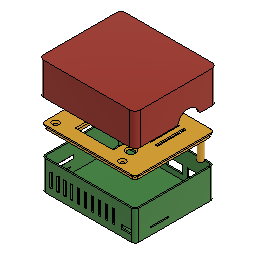
Raspi Zero 2W Case Battery V1 (Autodesk Fusion 360 design; units mm, degrees)
Autodesk Fusion 360 part; units mm, degrees
sketch "Skizze1" plane through (0, 0, 0) normal (0, 0, 1) x (1, 0, 0)
  line L0 (0, 0) -> (78.8, 0) construction
  line L1 (78.8, 0) -> (78.8, 62.5) construction
  line L2 (78.8, 62.5) -> (0, 62.5) construction
  line L3 (0, 62.5) -> (0, 0) construction
  line L4 (2, 65) -> (76.8, 65)
  line L5 (78.8, 63) -> (78.8, 0.5)
  line L6 (76.8, -1.5) -> (2, -1.5)
  line L7 (0, 0.5) -> (0, 63)
  circle A0 centre (75.3, 59) radius 1.5
  circle A1 centre (4.8, 59) radius 1.5
  circle A2 centre (4.8, 3.5) radius 1.5
  circle A3 centre (62.8, 3.5) radius 1.5
  circle A4 centre (4.8, 26.5) radius 1.5
  circle A5 centre (62.8, 26.5) radius 1.5
  circle A6 centre (4.8, 59) radius 2.5
  circle A7 centre (75.3, 59) radius 2.5
  circle A8 centre (4.8, 3.5) radius 2.5
  circle A9 centre (62.8, 3.5) radius 2.5
  arc A10 (78.8, 63) -> (76.8, 65) centre (76.8, 63) ccw
  arc A11 (2, 65) -> (0, 63) centre (2, 63) ccw
  arc A12 (0, 0.5) -> (2, -1.5) centre (2, 0.5) ccw
  arc A13 (76.8, -1.5) -> (78.8, 0.5) centre (76.8, 0.5) ccw
  line L8 (76.8, -2.7) -> (2, -2.7)
  arc A14 (-1.2, 0.5) -> (2, -2.7) centre (2, 0.5) ccw
  line L9 (-1.2, 0.5) -> (-1.2, 63)
  arc A15 (2, 66.2) -> (-1.2, 63) centre (2, 63) ccw
  line L10 (2, 66.2) -> (76.8, 66.2)
  arc A16 (80, 63) -> (76.8, 66.2) centre (76.8, 63) ccw
  line L11 (80, 63) -> (80, 0.5)
  arc A17 (76.8, -2.7) -> (80, 0.5) centre (76.8, 0.5) ccw
  dimension "d1" = 78.8
  dimension "d2" = 62.5
  dimension "d7" = 66.5
  dimension "d8" = 78.8
  dimension "d9" = 78.8
  dimension "d10" = 2.5
  dimension "d11" = 3
  dimension "d13" = 3.5
  dimension "d15" = 3
  dimension "d16" = 4.8
  dimension "d18" = 3.5
  dimension "d19" = 3.5
  dimension "d21" = 3
  dimension "d22" = 3.5
  dimension "d23" = 4.8
  dimension "d24" = 3
  dimension "d25" = 3.5
  dimension "d26" = 58
  dimension "d29" = 3
  dimension "d30" = 23
  dimension "d31" = 4.8
  dimension "d32" = 3
  dimension "d33" = 58
  dimension "d34" = 23
  dimension "d44" = 5
  dimension "d45" = 5
  dimension "d46" = 5
  dimension "d47" = 5
  dimension "d50" = 2
  dimension "d112" = 70.5
  constraint horizontal L0
  constraint vertical L1
  constraint horizontal L2
  constraint vertical L3
  constraint coincident L0.start L3.end
  constraint horizontal L4
  constraint vertical L5
  constraint horizontal L6
  constraint vertical L7
  constraint concentric A1 A6
  constraint concentric A0 A7
  constraint concentric A2 A8
  constraint concentric A3 A9
  constraint tangent L4 A10
  constraint tangent L5 A10
  constraint tangent L4 A11
  constraint tangent L7 A11
  constraint equal A10 A11
  constraint tangent L6 A12
  constraint tangent L7 A12
  constraint equal A10 A12
  constraint tangent L5 A13
  constraint tangent L6 A13
  constraint equal A10 A13
  measures "d1" distance of L0.start L0.end
  measures "d2" distance of L0.start L2.end
  measures "d7" distance of L4 L6
  measures "d8" distance of L5 L7
  measures "d9" distance of L3 L5
  measures "d10" distance of L2 L4
  measures "d11" diameter of A0
  measures "d13" distance of L5 A0.centre
  measures "d15" diameter of A1
  measures "d16" distance of L7 A1.centre
  measures "d18" distance of L2 A1.centre
  measures "d19" distance of L2 A0.centre
  measures "d21" diameter of A2
  measures "d22" distance of L0 A2.centre
  measures "d23" distance of L7 A2.centre
  measures "d24" diameter of A3
  measures "d25" distance of L0 A3.centre
  measures "d26" distance of A2.centre A3.centre
  measures "d29" diameter of A4
  measures "d30" vertical distance of A2.centre A4.centre
  measures "d31" distance of L7 A4.centre
  measures "d32" diameter of A5
  measures "d33" horizontal distance of A4.centre A5.centre
  measures "d34" distance of A3.centre A5.centre
  measures "d44" diameter of A6
  measures "d45" diameter of A7
  measures "d46" diameter of A8
  measures "d47" diameter of A9
  measures "d50" radius of A10
  measures "d112" distance of A1.centre A0.centre
extrude "Extrusion1" add sketch "Skizze1" against normal blind 1.2 contours L4 L5 L6 L7 A10 A11 A12 A13 | A0 | A1 | A2 | A3 | A4 | A5 | A6 | A7 | A8 | A9 | L8 A14 L9 A15 L10 A16 L11 A17 makes body 1
extrude "Extrusion2" add sketch "Skizze1" along normal blind 24.5 contours L8 A14 L9 A15 L10 A16 L11 A17 bodies 1
extrude "Extrusion3" add sketch "Skizze1" along normal blind 3 contours A6 | A7 | A8 | A9 bodies 1
extrude "Extrusion4" cut sketch "Skizze1" against normal blind 1.2 contours A0 | A1 | A2 | A3 bodies 1
chamfer "Fase1" distance 1.4 angle 45 4 edges at (61.4015, 2.9576, -1.2) (3.4015, 2.9576, -1.2) (3.4015, 58.4576, -1.2) (73.9015, 58.4576, -1.2) on bodies 1
ref_plane "Arbeitsebene1" through (82, 31.75, 11.65) normal (1, 0, 0) x (0, -1, 0)
sketch "Skizze2" plane through (82, 0, 0) normal (1, 0, 0) x (0, 1, 0)
  line L0 (11, 5.5) -> (26, 5.5)
  line L1 (26, 5.5) -> (26, 4.5)
  line L2 (26, 4.5) -> (11, 4.5)
  line L3 (11, 4.5) -> (11, 5.5)
  line L4 (7, 19.5) -> (8.5, 19.5)
  line L5 (8.5, 19.5) -> (8.5, 14.5)
  line L6 (8.5, 14.5) -> (7, 14.5)
  line L7 (7, 14.5) -> (7, 19.5)
  dimension "d65" = 15
  dimension "d66" = 1
  dimension "d68" = 11
  dimension "d69" = 4.5
  dimension "d109" = 1.5
  dimension "d110" = 5
  dimension "d111" = 14.5
  dimension "d119" = 7
  constraint horizontal L0
  constraint vertical L1
  constraint horizontal L2
  constraint vertical L3
  constraint horizontal L4
  constraint vertical L5
  constraint horizontal L6
  constraint vertical L7
  measures "d65" distance of L1 L3
  measures "d66" distance of L0 L2
  measures "d68" distance of origin L3
  measures "d69" distance of origin L2
  measures "d109" distance of L4.start L4.end
  measures "d110" distance of L4.start L6.end
  measures "d111" distance of origin L6
  measures "d119" distance of origin L7
extrude "Extrusion5" cut sketch "Skizze2" against normal blind 3.2 contours L0 L1 L2 L3 bodies 1
ref_plane "Arbeitsebene2" through (-3.2, 31.75, 11.65) normal (-1, 0, 0) x (0, 1, 0)
sketch "Skizze3" plane through (-3.2, 0, 0) normal (-1, 0, 0) x (0, -1, 0)
  line L0 (-21, 5.5) -> (-8, 5.5)
  line L1 (-8, 5.5) -> (-8, 4.5)
  line L2 (-8, 4.5) -> (-21, 4.5)
  line L3 (-21, 4.5) -> (-21, 5.5)
  line L4 (-63, 0) -> (-0.5, 0)
  line L5 (-24, 13) -> (-11, 13)
  line L6 (-11, 13) -> (-11, 10)
  line L7 (-11, 10) -> (-24, 10)
  line L8 (-24, 10) -> (-24, 13)
  dimension "d73" = 13
  dimension "d74" = 1
  dimension "d75" = 8
  dimension "d76" = 4.5
  dimension "d77" = 13
  dimension "d78" = 3
  dimension "d79" = 11
  dimension "d80" = 10
  constraint horizontal L0
  constraint vertical L1
  constraint horizontal L2
  constraint vertical L3
  constraint horizontal L5
  constraint vertical L6
  constraint horizontal L7
  constraint vertical L8
  measures "d73" distance of L0.start L0.end
  measures "d74" distance of L0 L2
  measures "d75" distance of origin L1
  measures "d76" distance of L2 L4
  measures "d77" distance of L6 L8
  measures "d78" distance of L5 L7
  measures "d79" distance of origin L6
  measures "d80" distance of L4 L7
extrude "Extrusion6" cut sketch "Skizze3" against normal blind 3.2 bodies 1
chamfer "Fase4" distance 1 angle 45 4 edges at (-1.2, 17.5, 13) (-1.2, 11, 11.5) (-1.2, 17.5, 10) (-1.2, 24, 11.5) on bodies 1
ref_plane "Arbeitsebene3" through (39.4, -4.7, 11.65) normal (0, -1, 0) x (-1, 0, 0)
sketch "Skizze4" plane through (0, -4.7, 0) normal (0, -1, 0) x (-1, 0, 0)
  line L0 (-76.8, -8) -> (-67.8, -8)
  line L1 (-67.8, -8) -> (-67.8, -4.5)
  line L2 (-67.8, -4.5) -> (-76.8, -4.5)
  line L3 (-76.8, -4.5) -> (-76.8, -8)
  line L4 (-6, -16.5) -> (-8, -16.5)
  line L5 (-8, -16.5) -> (-8, -4.5)
  line L6 (-8, -4.5) -> (-6, -4.5)
  line L7 (-6, -4.5) -> (-6, -16.5)
  line L8 (-12, -4.5) -> (-12, -16.5)
  line L9 (-14, -4.5) -> (-12, -4.5)
  line L10 (-14, -16.5) -> (-14, -4.5)
  line L11 (-12, -16.5) -> (-14, -16.5)
  line L12 (-18, -4.5) -> (-18, -16.5)
  line L13 (-20, -4.5) -> (-18, -4.5)
  line L14 (-20, -16.5) -> (-20, -4.5)
  line L15 (-18, -16.5) -> (-20, -16.5)
  line L16 (-24, -4.5) -> (-24, -16.5)
  line L17 (-26, -4.5) -> (-24, -4.5)
  line L18 (-26, -16.5) -> (-26, -4.5)
  line L19 (-24, -16.5) -> (-26, -16.5)
  line L20 (-30, -4.5) -> (-30, -16.5)
  line L21 (-32, -4.5) -> (-30, -4.5)
  line L22 (-32, -16.5) -> (-32, -4.5)
  line L23 (-30, -16.5) -> (-32, -16.5)
  line L24 (-36, -4.5) -> (-36, -16.5)
  line L25 (-38, -4.5) -> (-36, -4.5)
  line L26 (-38, -16.5) -> (-38, -4.5)
  line L27 (-36, -16.5) -> (-38, -16.5)
  line L28 (-42, -4.5) -> (-42, -16.5)
  line L29 (-44, -4.5) -> (-42, -4.5)
  line L30 (-44, -16.5) -> (-44, -4.5)
  line L31 (-42, -16.5) -> (-44, -16.5)
  line L32 (-48, -4.5) -> (-48, -16.5)
  line L33 (-50, -4.5) -> (-48, -4.5)
  line L34 (-50, -16.5) -> (-50, -4.5)
  line L35 (-48, -16.5) -> (-50, -16.5)
  line L36 (-54, -4.5) -> (-54, -16.5)
  line L37 (-56, -4.5) -> (-54, -4.5)
  line L38 (-56, -16.5) -> (-56, -4.5)
  line L39 (-54, -16.5) -> (-56, -16.5)
  line L40 (-60, -4.5) -> (-60, -16.5)
  line L41 (-62, -4.5) -> (-60, -4.5)
  line L42 (-62, -16.5) -> (-62, -4.5)
  line L43 (-60, -16.5) -> (-62, -16.5)
  dimension "d84" = 9
  dimension "d85" = 3.5
  dimension "d86" = 76.8
  dimension "d87" = 4.5
  dimension "d171" = 2
  dimension "d172" = 12
  dimension "d173" = 4.5
  dimension "d176" = -6
  dimension "d177" = 0
  dimension "d178" = 6
  constraint horizontal L0
  constraint vertical L1
  constraint horizontal L2
  constraint vertical L3
  constraint horizontal L4
  constraint vertical L5
  constraint horizontal L6
  constraint vertical L7
  measures "d84" distance of L0.start L0.end
  measures "d85" distance of L0 L2
  measures "d86" distance of origin L3
  measures "d87" distance of origin L2
  measures "d171" distance of L5 L7
  measures "d172" distance of L4 L6
  measures "d173" distance of origin L6
  measures "d178" distance of origin L7
extrude "Extrusion7" cut sketch "Skizze4" against normal blind 3.2 bodies 1
ref_plane "Arbeitsebene4" through (39.4, 68.2, 11.65) normal (0, 1, 0) x (1, 0, 0)
sketch "Skizze5" plane through (0, 68.2, 0) normal (0, 1, 0) x (1, 0, 0)
  line L0 (76.8, 0) -> (2, 0)
  line L1 (35.8, -11.5) -> (21.8, -11.5)
  line L2 (21.8, -11.5) -> (21.8, -4.5)
  line L3 (21.8, -4.5) -> (35.8, -4.5)
  line L4 (35.8, -4.5) -> (35.8, -11.5)
  line L5 (53.8, -11.5) -> (39.8, -11.5)
  line L6 (39.8, -11.5) -> (39.8, -4.5)
  line L7 (39.8, -4.5) -> (53.8, -4.5)
  line L8 (53.8, -4.5) -> (53.8, -11.5)
  line L9 (71.8, -11.5) -> (57.8, -11.5)
  line L10 (57.8, -11.5) -> (57.8, -4.5)
  line L11 (57.8, -4.5) -> (71.8, -4.5)
  line L12 (71.8, -4.5) -> (71.8, -11.5)
  line L13 (13.4, -13.3) -> (10.4, -13.3)
  line L14 (10.4, -13.3) -> (10.4, -3.3)
  line L15 (10.4, -3.3) -> (13.4, -3.3)
  line L16 (13.4, -3.3) -> (13.4, -13.3)
  line L17 (11.9, -49) -> (11.9, 25) construction
  line L18 (91, -8.3) -> (-18, -8.3) construction
  line L19 (-1.2, 1.2) -> (-1.2, -24.5)
  line L20 (2, 1.2) -> (76.8, 1.2)
  circle A0 centre (11.9, -8.3) radius 2.25
  dimension "d94" = 14
  dimension "d95" = 7
  dimension "d96" = 11.5
  dimension "d97" = 21.8
  dimension "d98" = 7
  dimension "d99" = 11.5
  dimension "d100" = 14
  dimension "d101" = 18
  dimension "d102" = 7
  dimension "d103" = 14
  dimension "d104" = 11.5
  dimension "d105" = 18
  dimension "d114" = 10
  dimension "d115" = 3
  dimension "d124" = 4.5
  dimension "d125" = 11.9
  dimension "d126" = 8.3
  constraint horizontal L1
  constraint vertical L2
  constraint horizontal L3
  constraint vertical L4
  constraint horizontal L5
  constraint vertical L6
  constraint horizontal L7
  constraint vertical L8
  constraint horizontal L9
  constraint vertical L10
  constraint horizontal L11
  constraint vertical L12
  constraint horizontal L13
  constraint vertical L14
  constraint horizontal L15
  constraint vertical L16
  constraint perpendicular L0 L17
  constraint perpendicular L6 L18
  constraint coincident L18 A0.centre
  constraint coincident L17 A0.centre
  constraint symmetric L13 L15 L18
  constraint symmetric L14 L16 L17
  measures "d94" distance of L1.start L1.end
  measures "d95" distance of L1.start L3.end
  measures "d96" distance of L0 L1
  measures "d97" distance of origin L2
  measures "d98" distance of L5 L7
  measures "d99" distance of L0 L5
  measures "d100" distance of L6 L8
  measures "d101" distance of L2 L6
  measures "d102" distance of L9 L11
  measures "d103" distance of L10 L12
  measures "d104" distance of L0 L9
  measures "d105" distance of L6 L10
  measures "d114" distance of L13 L15
  measures "d115" distance of L14 L16
  measures "d124" diameter of A0
  measures "d125" distance of origin L17
  measures "d126" distance of origin L18
extrude "Extrusion8" cut sketch "Skizze5" against normal blind 3.2 bodies 1
chamfer "Fase6" distance 1 angle 45 8 edges at (11.9, 66.2, 13.3) (10.4, 66.2, 11.6385) (9.65, 66.2, 8.3) (10.4, 66.2, 4.9615) (11.9, 66.2, 3.3) (13.4, 66.2, 4.9615) (14.15, 66.2, 8.3) (13.4, 66.2, 11.6385) on bodies 1
ref_plane "Arbeitsebene5" through (39.4, 31.75, 28.5) normal (0, 0, 1) x (1, 0, 0)
sketch "Skizze6" plane through (0, 0, 28.5) normal (0, 0, 1) x (1, 0, 0)
  arc A0 (0, 0.5) -> (2, -1.5) centre (2, 0.5) ccw construction
  line L0 (0, 0.5) -> (0, 63) construction
  arc A1 (2, 65) -> (0, 63) centre (2, 63) ccw construction
  line L1 (2, 65) -> (76.8, 65) construction
  arc A2 (78.8, 63) -> (76.8, 65) centre (76.8, 63) ccw construction
  line L2 (78.8, 63) -> (78.8, 0.5) construction
  arc A3 (76.8, -1.5) -> (78.8, 0.5) centre (76.8, 0.5) ccw construction
  line L3 (76.8, -1.5) -> (2, -1.5) construction
  arc A4 (-1.2, 0.5) -> (2, -2.7) centre (2, 0.5) ccw construction
  line L4 (2, -2.7) -> (76.8, -2.7) construction
  arc A5 (76.8, -2.7) -> (80, 0.5) centre (76.8, 0.5) ccw construction
  line L5 (80, 0.5) -> (80, 63) construction
  arc A6 (80, 63) -> (76.8, 66.2) centre (76.8, 63) ccw construction
  line L6 (76.8, 66.2) -> (2, 66.2) construction
  arc A7 (2, 66.2) -> (-1.2, 63) centre (2, 63) ccw construction
  line L7 (-1.2, 63) -> (-1.2, 0.5) construction
  circle A8 centre (4.8, 3.5) radius 1.5
  circle A9 centre (62.8, 3.5) radius 1.5
  circle A10 centre (75.3, 59) radius 1.5
  circle A11 centre (4.8, 59) radius 1.5
  arc A12 (2, 64.95) -> (0.05, 63) centre (2, 63) ccw
  line L8 (0.05, 0.5) -> (0.05, 63)
  arc A13 (0.05, 0.5) -> (2, -1.45) centre (2, 0.5) ccw
  line L9 (76.8, -1.45) -> (2, -1.45)
  arc A14 (76.8, -1.45) -> (78.75, 0.5) centre (76.8, 0.5) ccw
  line L10 (78.75, 63) -> (78.75, 0.5)
  arc A15 (78.75, 63) -> (76.8, 64.95) centre (76.8, 63) ccw
  line L11 (2, 64.95) -> (76.8, 64.95)
  arc A16 (2, 63.75) -> (1.25, 63) centre (2, 63) ccw
  line L12 (1.25, 0.5) -> (1.25, 63)
  arc A17 (1.25, 0.5) -> (2, -0.25) centre (2, 0.5) ccw
  line L13 (76.8, -0.25) -> (2, -0.25)
  arc A18 (76.8, -0.25) -> (77.55, 0.5) centre (76.8, 0.5) ccw
  line L14 (77.55, 63) -> (77.55, 0.5)
  arc A19 (77.55, 63) -> (76.8, 63.75) centre (76.8, 63) ccw
  line L15 (2, 63.75) -> (76.8, 63.75)
  arc A20 (2, 66.2) -> (-1.2, 63) centre (2, 63) ccw
  line L16 (-1.2, 0.5) -> (-1.2, 63)
  arc A21 (-1.2, 0.5) -> (2, -2.7) centre (2, 0.5) ccw
  line L17 (76.8, -2.7) -> (2, -2.7)
  arc A22 (76.8, -2.7) -> (80, 0.5) centre (76.8, 0.5) ccw
  line L18 (80, 63) -> (80, 0.5)
  arc A23 (80, 63) -> (76.8, 66.2) centre (76.8, 63) ccw
  line L19 (2, 66.2) -> (76.8, 66.2)
  circle A24 centre (4.8, 3.5) radius 2.5
  circle A25 centre (4.8, 59) radius 2.5
  circle A26 centre (75.3, 59) radius 2.5
  circle A27 centre (62.8, 3.5) radius 2.5
  circle A28 centre (58.55, 15.25) radius 3
  line L20 (18.3, 25) -> (49.3, 25)
  line L21 (49.3, 25) -> (49.3, 9)
  line L22 (49.3, 9) -> (18.3, 9)
  line L23 (18.3, 9) -> (18.3, 25)
  line L24 (50.5, 26.2) -> (50.5, 7.8)
  line L25 (50.5, 7.8) -> (17.1, 7.8)
  line L26 (17.1, 7.8) -> (17.1, 26.2)
  line L27 (17.1, 26.2) -> (50.5, 26.2)
  line L28 (10.8, 54.95) -> (12.8, 54.95)
  line L29 (12.8, 54.95) -> (12.8, 29.95)
  line L30 (12.8, 29.95) -> (10.8, 29.95)
  line L31 (10.8, 29.95) -> (10.8, 54.95)
  line L32 (16.8, 54.95) -> (18.8, 54.95)
  line L33 (16.8, 29.95) -> (16.8, 54.95)
  line L34 (18.8, 54.95) -> (18.8, 29.95)
  line L35 (18.8, 29.95) -> (16.8, 29.95)
  line L36 (22.8, 54.95) -> (24.8, 54.95)
  line L37 (22.8, 29.95) -> (22.8, 54.95)
  line L38 (24.8, 54.95) -> (24.8, 29.95)
  line L39 (24.8, 29.95) -> (22.8, 29.95)
  line L40 (28.8, 54.95) -> (30.8, 54.95)
  line L41 (28.8, 29.95) -> (28.8, 54.95)
  line L42 (30.8, 54.95) -> (30.8, 29.95)
  line L43 (30.8, 29.95) -> (28.8, 29.95)
  line L44 (34.8, 54.95) -> (36.8, 54.95)
  line L45 (34.8, 29.95) -> (34.8, 54.95)
  line L46 (36.8, 54.95) -> (36.8, 29.95)
  line L47 (36.8, 29.95) -> (34.8, 29.95)
  line L48 (40.8, 54.95) -> (42.8, 54.95)
  line L49 (40.8, 29.95) -> (40.8, 54.95)
  line L50 (42.8, 54.95) -> (42.8, 29.95)
  line L51 (42.8, 29.95) -> (40.8, 29.95)
  line L52 (46.8, 54.95) -> (48.8, 54.95)
  line L53 (46.8, 29.95) -> (46.8, 54.95)
  line L54 (48.8, 54.95) -> (48.8, 29.95)
  line L55 (48.8, 29.95) -> (46.8, 29.95)
  line L56 (52.8, 54.95) -> (54.8, 54.95)
  line L57 (52.8, 29.95) -> (52.8, 54.95)
  line L58 (54.8, 54.95) -> (54.8, 29.95)
  line L59 (54.8, 29.95) -> (52.8, 29.95)
  line L60 (58.8, 54.95) -> (60.8, 54.95)
  line L61 (58.8, 29.95) -> (58.8, 54.95)
  line L62 (60.8, 54.95) -> (60.8, 29.95)
  line L63 (60.8, 29.95) -> (58.8, 29.95)
  line L64 (64.8, 54.95) -> (66.8, 54.95)
  line L65 (64.8, 29.95) -> (64.8, 54.95)
  line L66 (66.8, 54.95) -> (66.8, 29.95)
  line L67 (66.8, 29.95) -> (64.8, 29.95)
  circle A29 centre (75.3, 59) radius 1.2
  circle A30 centre (4.8, 59) radius 1.2
  dimension "d130" = 0.05
  dimension "d131" = 1.25
  dimension "d143" = 6
  dimension "d144" = 11.75
  dimension "d145" = 4.25
  dimension "d149" = 31
  dimension "d150" = 16
  dimension "d151" = 5.5
  dimension "d152" = 13.5
  dimension "d159" = 10
  dimension "d160" = 10.75
  dimension "d163" = 6
  dimension "d164" = 0
  dimension "d165" = 56
  dimension "d179" = 2.4
  dimension "d180" = 2.4
  constraint horizontal L20
  constraint vertical L21
  constraint horizontal L22
  constraint vertical L23
  constraint horizontal L28
  constraint vertical L29
  constraint horizontal L30
  constraint vertical L31
  constraint concentric A10 A29
  constraint concentric A11 A30
  measures "d143" diameter of A28
  measures "d144" vertical distance of A9.centre A28.centre
  measures "d145" horizontal distance of A9.centre A28.centre
  measures "d149" distance of L20.start L20.end
  measures "d150" distance of L20.start L22.end
  measures "d151" distance of A9.centre L22
  measures "d152" distance of A9.centre L21
  measures "d159" distance of L11 L28
  measures "d160" distance of L8 L31
  measures "d165" distance of L31 L66
  measures "d179" diameter of A29
  measures "d180" diameter of A30
extrude "Extrusion9" add sketch "Skizze6" along normal blind 1.2 separate body contours A8 | A9 | A10 | A11 | A12 L8 A13 L9 A14 L10 A15 L11 | A16 L12 A17 L13 A18 L14 A19 L15 A26 | L14 A26 | L14 A26 | A20 L16 A21 L17 A22 L18 A23 L19 | A24 | A25 | A27 | A28 | L20 L21 L22 L23 | L24 L25 L26 L27 | L28 L29 L30 L31 | L32 L33 L34 L35 | L36 L37 L38 L39 | L40 L41 L42 L43 | L44 L45 L46 L47 | L48 L49 L50 L51 | L52 L53 L54 L55 | L56 L57 L58 L59 | L60 L61 L62 L63 | L64 L65 L66 L67 | A29 | A30 makes body 2
extrude "Extrusion10" add sketch "Skizze6" against normal blind 3 contours A12 L8 A13 L9 A14 L10 A15 L11 | L14 A26 picked at (77.5861, 58.7235) bodies 2
extrude "Extrusion11" cut sketch "Skizze6" along normal blind 1.2 contours A8 | A9 bodies 2
extrude "Extrusion12" add sketch "Skizze6" against normal blind 3.5 contours A10 | A11 | L14 A26 | A24 | A25 | A27 | A29 | A30 picked at (77.3, 59) bodies 2
chamfer "Fase7" distance 1.4 angle 45 2 edges at (3.4015, 4.0424, 29.7) (61.4015, 4.0424, 29.7) on bodies 2
extrude "Extrusion13" cut sketch "Skizze6" along normal blind 1.2 contours A28 bodies 2
chamfer "Fase8" distance 1 angle 45 1 edges at (55.753, 16.3348, 29.7) on bodies 2
extrude "Extrusion14" cut sketch "Skizze6" along normal blind 1.2 contours L20 L21 L22 L23 bodies 2
chamfer "Fase9" distance 1 angle 45 4 edges at (18.3, 17, 29.7) (33.8, 25, 29.7) (49.3, 17, 29.7) (33.8, 9, 29.7) on bodies 2
extrude "Extrusion15" add sketch "Skizze6" against normal blind 2 contours L24 L25 L26 L27 bodies 2
extrude "Extrusion16" cut sketch "Skizze6" along normal blind 1.2 contours L28 L29 L30 L31 | L32 L33 L34 L35 | L36 L37 L38 L39 | L40 L41 L42 L43 | L44 L45 L46 L47 | L48 L49 L50 L51 | L52 L53 L54 L55 | L56 L57 L58 L59 | L60 L61 L62 L63 | L64 L65 L66 L67 bodies 2
extrude "Extrusion17" add sketch "Skizze6" against normal blind 19.5 contours A10 | A11 | L14 A26 | L14 A26 | A25 bodies 2
ref_plane "Arbeitsebene6" through (39.4, 31.75, 59.8) normal (0, 0, 1) x (1, 0, 0)
sketch "Skizze7" plane through (0, 0, 59.8) normal (0, 0, 1) x (1, 0, 0)
  line L0 (-1.2, 0.5) -> (-1.2, 63) construction
  arc A0 (2, 66.2) -> (-1.2, 63) centre (2, 63) ccw construction
  line L1 (2, 66.2) -> (76.8, 66.2) construction
  arc A1 (80, 63) -> (76.8, 66.2) centre (76.8, 63) ccw construction
  line L2 (80, 63) -> (80, 0.5) construction
  arc A2 (76.8, -2.7) -> (80, 0.5) centre (76.8, 0.5) ccw construction
  line L3 (76.8, -2.7) -> (2, -2.7) construction
  arc A3 (-1.2, 0.5) -> (2, -2.7) centre (2, 0.5) ccw construction
  arc A4 (-1.25, 0.5) -> (2, -2.75) centre (2, 0.5) ccw
  line L4 (76.8, -2.75) -> (2, -2.75)
  arc A5 (76.8, -2.75) -> (80.05, 0.5) centre (76.8, 0.5) ccw
  line L5 (80.05, 63) -> (80.05, 0.5)
  arc A6 (80.05, 63) -> (76.8, 66.25) centre (76.8, 63) ccw
  line L6 (2, 66.25) -> (76.8, 66.25)
  arc A7 (2, 66.25) -> (-1.25, 63) centre (2, 63) ccw
  line L7 (-1.25, 0.5) -> (-1.25, 63)
  arc A8 (2, 67.45) -> (-2.45, 63) centre (2, 63) ccw
  line L8 (-2.45, 0.5) -> (-2.45, 63)
  arc A9 (-2.45, 0.5) -> (2, -3.95) centre (2, 0.5) ccw
  line L9 (76.8, -3.95) -> (2, -3.95)
  arc A10 (76.8, -3.95) -> (81.25, 0.5) centre (76.8, 0.5) ccw
  line L10 (81.25, 63) -> (81.25, 0.5)
  arc A11 (81.25, 63) -> (76.8, 67.45) centre (76.8, 63) ccw
  line L11 (2, 67.45) -> (76.8, 67.45)
  dimension "d185" = 0.05
extrude "Extrusion18" add sketch "Skizze7" against normal blind 26.9 separate body makes body 3
ref_plane "Arbeitsebene7" through (83.25, 31.75, 46.35) normal (1, 0, 0) x (0, -1, 0)
sketch "Skizze8" plane through (83.25, 0, 0) normal (1, 0, 0) x (0, 1, 0)
  line L0 (67.45, 59.8) -> (67.45, 32.9)
  line L1 (63, 32.9) -> (0.5, 32.9)
  circle A0 centre (42.45, 31.9) radius 9.25
  line L2 (63, 59.8) -> (0.5, 59.8)
  point P0 (-3.95, 32.9)
  point P1 (67.45, 32.9)
  dimension "d191" = 71.4
  dimension "d196" = 18.5
  dimension "d197" = 25
  dimension "d198" = 27.9
  dimension "d199" = 26.9
  measures "d191" distance of P0 L0.end
  measures "d196" diameter of A0
  measures "d197" distance of L0 A0.centre
  measures "d198" distance of A0.centre L2
  measures "d199" distance of L1 L2
extrude "Extrusion19" cut sketch "Skizze8" against normal blind 85.7 contours L1 A0 picked at (41.1402, 37.0973) bodies 3
extrude "Extrusion20" add sketch "Skizze7" along normal blind 1.2 contours A4 L4 A5 L5 A6 L6 A7 L7 | A8 L8 A9 L9 A10 L10 A11 L11 bodies 3
fillet "Abrundung1" radius 2 4 edges at (80.65, 51.6458, 32.9) (80.65, 33.2542, 32.9) (-1.85, 33.2542, 32.9) (-1.85, 51.6458, 32.9) on bodies 3
copy_body "Körper->Berechn1" bodies 1 removing the originals makes body 4 in component "bottom_Zero2W_battery_case"
copy_body "Körper->Berechn2" bodies 2 removing the originals makes body 5 in component "top_Zero2W_battery_case"
copy_body "Körper->Berechn3" bodies 3 removing the originals makes body 6 in component "cover_Zero2W_battery_case"
move_body "Verschieben1" bodies 6 to x (1, 0, 0) y (0, 1, 0) z (0, 0, 1) at (0, 0, 38) in component "cover_Zero2W_battery_case"
move_body "Verschieben1'" bodies 5 to x (1, 0, 0) y (0, 1, 0) z (0, 0, 1) at (0, 0, 20) in component "top_Zero2W_battery_case"
component "bottom_Zero2W_battery_case" placed x (1, 0, 0) y (0, 1, 0) z (0, 0, 1) at (0, 0, 0)
component "top_Zero2W_battery_case" placed x (1, 0, 0) y (0, 1, 0) z (0, 0, 1) at (0, 0, 0)
component "cover_Zero2W_battery_case" placed x (1, 0, 0) y (0, 1, 0) z (0, 0, 1) at (0, 0, 0)
equation "d1 = board_laenge + sd_add"
equation "d2 = board_breite"
equation "board_laenge = 77.5 mm"
equation "board_breite = 62.5 mm"
equation "usba_add = 2.5 mm"
equation "usbc_add = 1.5 mm"
equation "d7 = d2 + usba_add + usbc_add"
equation "d8 = d1"
equation "d9 = d1"
equation "d10 = usba_add"
equation "d11 = board_bohrung"
equation "board_bohrung = 3 mm"
equation "d15 = d11"
equation "d16 = d13 + sd_add"
equation "d18 = d19"
equation "knopf_add = 5 mm"
equation "d21 = board_bohrung"
equation "d22 = d13"
equation "d23 = d16"
equation "d24 = board_bohrung"
equation "d25 = d13"
equation "d26 = zero_loch_laenge"
equation "zero_loch_breit = 23 mm"
equation "zero_loch_laenge = 58 mm"
equation "d29 = board_bohrung"
equation "d30 = zero_loch_breit"
equation "d31 = d16"
equation "d32 = board_bohrung"
equation "d33 = zero_loch_laenge"
equation "d34 = zero_loch_breit"
equation "wanddicke = 1.2 mm"
equation "abstand_boden = 3 mm"
equation "d37 = -wanddicke"
equation "d38 = -wanddicke"
equation "d40 = abstand_boden + board_hoehe"
equation "board_hoehe = 21.5 mm"
equation "abstand_durchmesser = 5 mm"
equation "d44 = abstand_durchmesser"
equation "d45 = d44"
equation "d46 = d44"
equation "d47 = d44"
equation "d48 = abstand_boden"
equation "d50 = board_radius"
equation "board_radius = 2 mm"
equation "d52 = -wanddicke"
equation "d54 = schrauben_fase"
equation "schrauben_fase = 1.4 mm"
equation "board_dicke = 1.5 mm"
equation "b_schlitz_hoehe = 1 mm"
equation "b_schlitz_breite = 15 mm"
equation "b_schlitz_abstand = 11 mm"
equation "r_schlitz_hoehe = 1 mm"
equation "r_schlitz_breite = 13 mm"
equation "r_schlitz_abstand = 8 mm"
equation "abstand_ebene = 2 mm"
equation "d64 = abstand_ebene"
equation "d65 = b_schlitz_breite"
equation "d66 = b_schlitz_hoehe"
equation "d68 = b_schlitz_abstand"
equation "d69 = abstand_boden + board_dicke"
equation "d70 = -( abstand_ebene + wanddicke )"
equation "d72 = abstand_ebene"
equation "d73 = r_schlitz_breite"
equation "d74 = r_schlitz_hoehe"
equation "d75 = r_schlitz_abstand"
equation "d76 = abstand_boden + board_dicke"
equation "d80 = abstand_boden + 7 mm"
equation "d81 = -( abstand_ebene + wanddicke )"
equation "d83 = abstand_ebene"
equation "d86 = board_laenge - 2 mm + sd_add"
equation "d87 = abstand_boden + board_dicke"
equation "d88 = -( abstand_ebene + wanddicke )"
equation "d90 = abstand_ebene"
equation "d96 = 7 mm + abstand_boden + board_dicke"
equation "d97 = 20.5 mm + sd_add"
equation "d98 = d95"
equation "d99 = d96"
equation "d100 = d94"
equation "d102 = d95"
equation "d103 = d94"
equation "d104 = d96"
equation "d105 = d101"
equation "d106 = -( abstand_ebene + wanddicke )"
equation "d111 = 10 mm + abstand_boden + board_dicke"
equation "sd_add = 1.3 mm"
equation "d125 = sd_add + 10.6 mm"
equation "d128 = 2 * abstand_ebene"
equation "gap = 0.05 mm"
equation "d130 = gap"
equation "d131 = gap + wanddicke"
equation "d132 = -wanddicke"
equation "d133 = wanddicke"
equation "d137 = wanddicke"
equation "d139 = -abstand_deckel"
equation "abstand_deckel = 3.5 mm"
equation "d142 = schrauben_fase"
equation "d146 = wanddicke"
equation "d153 = wanddicke"
equation "d156 = -wanddicke"
equation "d160 = ( board_laenge - d165 ) / 2"
equation "d166 = wanddicke"
equation "breite_lueftung = 2 mm"
equation "d171 = breite_lueftung"
equation "d173 = d87"
equation "d176 = -3 * breite_lueftung"
equation "gehaeuse_hoehe = board_hoehe + abstand_boden + wanddicke * 2"
equation "gehaeuse_breite = board_breite + usba_add + usbc_add + wanddicke * 2"
equation "gehaeuse_laenge = board_laenge + sd_add + wanddicke * 2"
equation "d184 = abstand_ebene + gehaeuse_hoehe + wanddicke"
equation "d185 = gap"
equation "d186 = -( gap + wanddicke )"
equation "d187 = -( gehaeuse_hoehe )"
equation "d189 = abstand_ebene"
equation "d198 = d199 + 1 mm"
equation "d200 = -( abstand_ebene + wanddicke + gehaeuse_laenge + wanddicke + gap * 2 )"
equation "d202 = wanddicke"
named bodies: "bottom_Zero2W_battery_case", "top_Zero2W_battery_case", "cover_Zero2W_battery_case"
